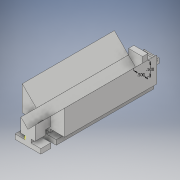
# Autodesk Inventor part: structureholder
Saved by Autodesk Inventor 2018 (Build 220112000, 112)
## iProperties
Created: 2019-02-25
Part Number: structureholder
Material: Generic
Document SubType Name: Modeling
Designer: F8PLTW
Density: 1 g/cm^3
Appearance: Default
Author: F8PLTW
Autodesk Inventor part; units mm, degrees
ref_plane "YZ Plane" through (0, 0, 0) normal (1, 0, 0) x (0, 1, 0)
ref_plane "XZ Plane" through (0, 0, 0) normal (0, 1, 0) x (-1, 0, 0)
ref_plane "XY Plane" through (0, 0, 0) normal (0, 0, 1) x (1, 0, 0)
sketch "Sketch1" plane through (0, 0, 0) normal (0, 0, 1) x (1, 0, 0)
  line L0 (-11.300905, 6.75881) -> (1.399095, 6.75881)
  line L1 (1.399095, 6.75881) -> (1.399095, -5.94119)
  line L2 (1.399095, -5.94119) -> (-11.300905, -5.94119)
  line L3 (-11.300905, -5.94119) -> (-11.300905, 6.75881)
  line L4 (-11.300905, 6.75881) -> (-1.742504, 6.75881) construction
  line L5 (-11.300905, 6.75881) -> (-4.950905, 0.40881)
  line L6 (1.399095, 6.75881) -> (-4.950905, 0.40881)
  point P0 (0, 0)
  dimension "d0" = 12.7
  dimension "d1" = 12.7
  constraints: 14 end point, 2 horizontal, 2 parallel, 1 perpendicular
  measures "d0" distance of L1.end L2.end
  measures "d1" distance of L0.end L1.end
sketch "Sketch1 outline for Extrusion1" plane through (0, 0, 0) normal (0, 0, 1) x (1, 0, 0)
  line L0 (-4.950905, 0.40881) -> (-11.300905, 6.75881)
  line L1 (1.399095, 6.75881) -> (-4.950905, 0.40881)
  line L2 (1.399095, -5.94119) -> (1.399095, 6.75881)
  line L3 (-11.300905, -5.94119) -> (1.399095, -5.94119)
  line L4 (-11.300905, 6.75881) -> (-11.300905, -5.94119)
extrude "Extrusion1" add sketch "Sketch1 outline for Extrusion1" along normal blind 101.6
sketch "Sketch1 outline for Extrusion2" plane through (0, 0, 0) normal (0, 0, 1) x (1, 0, 0)
  line L0 (1.399095, 6.75881) -> (-11.300905, 6.75881)
  line L1 (-4.950905, 0.40881) -> (1.399095, 6.75881)
  line L2 (-11.300905, 6.75881) -> (-4.950905, 0.40881)
extrude "Extrusion2" add sketch "Sketch1 outline for Extrusion2" along normal blind 5.08
sketch "Sketch2" plane through (-11.300905, 6.75881, 0) normal (0, 1, 0) x (1, 0, 0)
  line L0 (0, 0) -> (0, -101.6)
  line L1 (12.7, 0) -> (12.7, -101.6)
  line L2 (0, 0) -> (12.7, 0)
  line L3 (12.7, 0) -> (12.7, -5.078457)
  line L4 (12.7, -5.078457) -> (0, -5.078457)
  line L5 (0, -5.078457) -> (0, 0)
  point P0 (11.300905, 0)
  constraints: 8 end point, 2 parallel, 1 horizontal, 1 perpendicular, 1 point on line
sketch "Sketch2 outline for Extrusion3" plane through (-11.300905, 6.75881, 0) normal (0, 1, 0) x (1, 0, 0)
  line L0 (0, 0) -> (12.7, 0)
  line L1 (12.7, 0) -> (12.7, -5.078457)
  line L2 (12.7, -5.078457) -> (0, -5.078457)
  line L3 (0, -5.078457) -> (0, 0)
extrude "Extrusion3" add sketch "Sketch2 outline for Extrusion3" along normal blind 5.08
sketch "Sketch3" plane through (-11.300905, -5.94119, 0) normal (0, -1, 0) x (1, 0, 0)
  line L0 (12.7, 101.6) -> (6.35, 101.6) projected
  line L1 (0, 0) -> (12.7, 0) projected
  line L2 (9.4615, 101.6) -> (3.2385, 101.6)
  line L3 (3.2385, 101.6) -> (3.2385, 0)
  line L4 (3.2385, 0) -> (9.4615, 0)
  line L5 (9.4615, 0) -> (9.4615, 101.6)
  line L6 (6.35, 5.08) -> (6.35, 101.6) construction
  point P0 (11.300905, 0)
  dimension "d9" = 6.223
  constraints: 8 end point, 2 parallel, 2 point on line, 1 horizontal, 1 perpendicular, 1 other
  measures "d9" distance of L4.end L3.end
sketch "Sketch3 outline for Extrusion4" plane through (-11.300905, -5.94119, 0) normal (0, -1, 0) x (1, 0, 0)
  line L0 (9.4615, 0) -> (9.4615, 101.6)
  line L1 (3.2385, 0) -> (9.4615, 0)
  line L2 (3.2385, 101.6) -> (3.2385, 0)
  line L3 (9.4615, 101.6) -> (3.2385, 101.6)
extrude "Extrusion4" add sketch "Sketch3 outline for Extrusion4" along normal blind 7.3914
sketch "Sketch4" plane through (-1.839405, -5.94119, 101.6) normal (1, 0, 0) x (0, 0, -1)
  line L0 (101.6, -7.3914) -> (0, -7.3914) projected
  line L1 (101.6, 0) -> (101.6, -7.3914) projected
  line L2 (0, -7.3914) -> (101.6, -7.3914)
  line L3 (101.6, -7.3914) -> (101.6, -2.4384)
  line L4 (101.6, -2.4384) -> (0, -2.4384)
  line L5 (0, -2.4384) -> (0, -7.3914)
  point P0 (101.6, 5.94119)
  dimension "d12" = 4.953
  constraints: 8 end point, 2 parallel, 1 horizontal, 1 perpendicular, 1 point on line
  measures "d12" distance of L3.end L2.end
sketch "Sketch5" plane through (-8.062405, -5.94119, 0) normal (-1, 0, 0) x (0, 0, 1)
  line L0 (0, -7.3914) -> (101.6, -7.3914) projected
  line L1 (0, 0) -> (0, -7.3914) projected
  line L2 (101.6, -7.3914) -> (0, -7.3914)
  line L3 (0, -7.3914) -> (0, -2.4384)
  line L4 (0, -2.4384) -> (101.6, -2.4384)
  line L5 (101.6, -2.4384) -> (101.6, -7.3914)
  point P0 (0, 5.94119)
  dimension "d13" = 4.953
  constraints: 8 end point, 2 parallel, 1 horizontal, 1 perpendicular, 1 point on line
  measures "d13" distance of L2.end L3.end
sketch "Sketch5 outline for Extrusion5" plane through (-8.062405, -5.94119, 0) normal (-1, 0, 0) x (0, 0, 1)
  line L0 (0, -7.3914) -> (101.6, -7.3914)
  line L1 (0, -2.4384) -> (0, -7.3914)
  line L2 (101.6, -2.4384) -> (0, -2.4384)
  line L3 (101.6, -7.3914) -> (101.6, -2.4384)
extrude "Extrusion5" add sketch "Sketch5 outline for Extrusion5" along normal blind 8.763
sketch "Sketch4 outline for Extrusion6" plane through (-1.839405, -5.94119, 101.6) normal (1, 0, 0) x (0, 0, -1)
  line L0 (101.6, -7.3914) -> (101.6, -2.4384)
  line L1 (0, -7.3914) -> (101.6, -7.3914)
  line L2 (0, -2.4384) -> (0, -7.3914)
  line L3 (101.6, -2.4384) -> (0, -2.4384)
extrude "Extrusion6" add sketch "Sketch4 outline for Extrusion6" along normal blind 8.763
sketch "Sketch6" plane through (0, 0, 0) normal (0, 0, -1) x (-1, 0, 0)
  line L0 (-1.399095, -5.94119) -> (-1.399095, 6.75881)
  line L1 (-1.399095, 1.59881) -> (11.455496, 1.59881)
  line L2 (11.455496, 1.59881) -> (11.455496, -0.94119)
  line L3 (11.455496, -0.94119) -> (-1.399095, -0.94119)
  line L4 (-1.399095, -0.94119) -> (-1.399095, 1.59881)
  line L5 (11.300905, -5.94119) -> (8.062405, -5.94119)
  point P0 (0, 0)
  dimension "d18" = 2.54
  dimension "d19" = 5
  constraints: 8 end point, 2 parallel, 1 horizontal, 1 perpendicular, 1 point on line
  measures "d18" distance between parallel lines of L3 L1
  measures "d19" distance between parallel lines of L5 L3
sketch "Sketch6 outline for Extrusion7" plane through (0, 0, 0) normal (0, 0, -1) x (-1, 0, 0)
  line L0 (-1.399095, 1.59881) -> (11.455496, 1.59881)
  line L1 (11.455496, 1.59881) -> (11.455496, -0.94119)
  line L2 (11.455496, -0.94119) -> (-1.399095, -0.94119)
  line L3 (-1.399095, -0.94119) -> (-1.399095, 1.59881)
extrude "Extrusion7" add sketch "Sketch6 outline for Extrusion7" along normal blind 10
sketch "Sketch7" plane through (-11.300905, 1.59881, 0) normal (0, 1, 0) x (1, 0, 0)
  line L0 (-0.154591, 0) -> (-0.154591, 10)
  line L1 (12.7, 0) -> (12.7, 10)
  line L2 (-0.154591, 10) -> (12.7, 10)
  line L3 (12.7, 10) -> (12.7, 8.73819)
  line L4 (12.7, 8.73819) -> (-0.154591, 8.73819)
  line L5 (-0.154591, 8.73819) -> (-0.154591, 10)
  point P0 (11.300905, 0)
  constraints: 8 end point, 2 parallel, 1 horizontal, 1 perpendicular, 1 point on line
sketch "Sketch7 outline for Extrusion8" plane through (-11.300905, 1.59881, 0) normal (0, 1, 0) x (1, 0, 0)
  line L0 (-0.154591, 10) -> (12.7, 10)
  line L1 (12.7, 10) -> (12.7, 8.73819)
  line L2 (12.7, 8.73819) -> (-0.154591, 8.73819)
  line L3 (-0.154591, 8.73819) -> (-0.154591, 10)
extrude "Extrusion8" add sketch "Sketch7 outline for Extrusion8" along normal blind 2.5
fillet "Fillet1" radius 0.79375 2 edges at (-5.0282, 4.0988, -10) (-5.0282, 4.0988, -8.7382)
sketch "Sketch8" plane through (-11.300905, -13.33259, 0) normal (0, -1, 0) x (1, 0, 0)
  line L0 (18.2245, 101.6) -> (18.2245, 0)
  line L1 (-5.5245, 0) -> (-5.5245, 101.6)
  line L2 (18.2245, 92.457351) -> (-5.5245, 92.457351)
  line L3 (-5.5245, 92.457351) -> (-5.5245, 87.694851)
  line L4 (-5.5245, 87.694851) -> (18.2245, 87.694851)
  line L5 (18.2245, 87.694851) -> (18.2245, 92.457351)
  point P0 (11.300905, 0)
  dimension "d25" = 4.7625
  constraints: 8 end point, 2 parallel, 2 point on line, 1 horizontal, 1 perpendicular
  measures "d25" distance of L3.end L2.end
sketch "Sketch8 outline for Extrusion9" plane through (-11.300905, -13.33259, 0) normal (0, -1, 0) x (1, 0, 0)
  line L0 (18.2245, 87.694851) -> (18.2245, 92.457351)
  line L1 (-5.5245, 87.694851) -> (18.2245, 87.694851)
  line L2 (-5.5245, 92.457351) -> (-5.5245, 87.694851)
  line L3 (18.2245, 92.457351) -> (-5.5245, 92.457351)
extrude "Extrusion9" cut sketch "Sketch8 outline for Extrusion9" against normal blind 13.97
sketch "Sketch9" plane through (-11.300905, -13.33259, 0) normal (0, -1, 0) x (1, 0, 0)
  line L0 (-5.5245, 101.6) -> (18.2245, 101.6) projected
  line L1 (3.2385, 0) -> (-5.5245, 0) projected
  line L2 (18.2245, 101.6) -> (-5.5245, 101.6)
  line L3 (-5.5245, 101.6) -> (-5.5245, 0)
  line L4 (-5.5245, 0) -> (18.2245, 0)
  line L5 (18.2245, 0) -> (18.2245, 101.6)
  point P0 (11.300905, 0)
  constraints: 8 end point, 2 parallel, 1 horizontal, 1 perpendicular
sketch "Sketch9 outline for Extrusion10" plane through (-11.300905, -13.33259, 0) normal (0, -1, 0) x (1, 0, 0)
  line L0 (18.2245, 0) -> (18.2245, 101.6)
  line L1 (-5.5245, 0) -> (18.2245, 0)
  line L2 (-5.5245, 101.6) -> (-5.5245, 0)
  line L3 (18.2245, 101.6) -> (-5.5245, 101.6)
extrude "Extrusion10" cut sketch "Sketch9 outline for Extrusion10" against normal blind 0.127
sketch "Sketch10" plane through (-1.839405, -5.94119, 101.6) normal (0, -1, 0) x (1, 0, 0)
  line L0 (3.2385, -9.142649) -> (3.2385, 0)
  line L1 (0, -13.905149) -> (0, -101.6)
  line L2 (3.2385, 0) -> (0, 0)
  line L3 (0, 0) -> (0, -101.6)
  line L4 (0, -101.6) -> (3.2385, -101.6)
  line L5 (3.2385, -101.6) -> (3.2385, 0)
  line L6 (-9.4615, -9.142649) -> (-9.4615, 0)
  line L7 (-9.4615, -101.6) -> (3.2385, -101.6)
  line L8 (-9.4615, 0) -> (-5.941969, 0)
  line L9 (-5.941969, 0) -> (-5.941969, -101.6)
  line L10 (-5.941969, -101.6) -> (-9.4615, -101.6)
  line L11 (-9.4615, -101.6) -> (-9.4615, 0)
  point P0 (1.839405, -101.6)
  constraints: 16 end point, 4 parallel, 2 horizontal, 2 perpendicular, 1 point on line
sketch "Sketch10 outline for Extrusion11" plane through (-1.839405, -5.94119, 101.6) normal (0, -1, 0) x (1, 0, 0)
  line L0 (3.2385, -101.6) -> (3.2385, 0)
  line L1 (0, -101.6) -> (3.2385, -101.6)
  line L2 (0, 0) -> (0, -101.6)
  line L3 (3.2385, 0) -> (0, 0)
  line L4 (-9.4615, -101.6) -> (-5.941969, -101.6)
  line L5 (-9.4615, 0) -> (-9.4615, -101.6)
  line L6 (-5.941969, 0) -> (-9.4615, 0)
  line L7 (-5.941969, -101.6) -> (-5.941969, 0)
extrude "Extrusion11" cut sketch "Sketch10 outline for Extrusion11" against normal blind 0.127
sketch "Sketch11" plane through (6.923595, -5.94119, 101.6) normal (1, 0, 0) x (0, 0, -1)
  line L0 (0, -2.4384) -> (9.142649, -2.4384)
  line L1 (0, -2.4384) -> (101.6, -2.4384)
  line L2 (101.6, -2.4384) -> (101.6, -7.2644)
  line L3 (101.6, -7.2644) -> (0, -7.2644)
  line L4 (0, -7.2644) -> (0, -2.4384)
  point P0 (101.6, 5.94119)
  constraints: 8 end point, 2 parallel, 1 horizontal, 1 perpendicular
sketch "Sketch11 outline for Extrusion12" plane through (6.923595, -5.94119, 101.6) normal (1, 0, 0) x (0, 0, -1)
  line L0 (0, -2.4384) -> (101.6, -2.4384)
  line L1 (101.6, -2.4384) -> (101.6, -7.2644)
  line L2 (101.6, -7.2644) -> (0, -7.2644)
  line L3 (0, -7.2644) -> (0, -2.4384)
extrude "Extrusion12" cut sketch "Sketch11 outline for Extrusion12" against normal blind 0.0635
sketch "Sketch12" plane through (-16.825405, -5.94119, 0) normal (-1, 0, 0) x (0, 0, 1)
  line L0 (101.6, -7.2644) -> (101.6, -2.4384) projected
  line L1 (0, 0) -> (0, -2.4384) projected
  line L2 (101.6, -7.2644) -> (0, -7.2644)
  line L3 (0, -7.2644) -> (0, -2.4384)
  line L4 (0, -2.4384) -> (101.6, -2.4384)
  line L5 (101.6, -2.4384) -> (101.6, -7.2644)
  point P0 (0, 5.94119)
  constraints: 8 end point, 2 parallel, 1 horizontal, 1 perpendicular
sketch "Sketch12 outline for Extrusion13" plane through (-16.825405, -5.94119, 0) normal (-1, 0, 0) x (0, 0, 1)
  line L0 (101.6, -7.2644) -> (0, -7.2644)
  line L1 (0, -7.2644) -> (0, -2.4384)
  line L2 (0, -2.4384) -> (101.6, -2.4384)
  line L3 (101.6, -2.4384) -> (101.6, -7.2644)
extrude "Extrusion13" cut sketch "Sketch12 outline for Extrusion13" against normal blind 0.0635
sketch "Sketch13" plane through (-7.781374, -5.94119, 92.457351) normal (-1, 0, 0) x (0, 0, 1)
  line L0 (-92.457351, 0.127) -> (-4.7625, 0.127)
  line L1 (9.142649, -2.4384) -> (9.142649, 0.127)
  line L2 (-92.457351, 0.127) -> (9.142649, 0.127)
  line L3 (9.142649, 0.127) -> (9.142649, 0.002557)
  line L4 (9.142649, 0.002557) -> (-92.457351, 0.002557)
  line L5 (-92.457351, 0.002557) -> (-92.457351, 0.127)
  point P0 (-92.457351, 5.94119)
  constraints: 8 end point, 2 parallel, 1 horizontal, 1 perpendicular, 1 point on line
sketch "Sketch14" plane through (-7.781374, -5.94119, 0) normal (-1, 0, 0) x (0, 0, 1)
  line L0 (0, 0.127) -> (87.694851, 0.127)
  line L1 (92.457351, 0) -> (101.6, 0)
  line L2 (0, 0.127) -> (101.6, 0.127)
  line L3 (101.6, 0.127) -> (101.6, 0)
  line L4 (101.6, 0) -> (0, 0)
  line L5 (0, 0) -> (0, 0.127)
  point P0 (0, 5.94119)
  constraints: 8 end point, 2 parallel, 1 horizontal, 1 perpendicular
sketch "Sketch14 outline for Extrusion14" plane through (-7.781374, -5.94119, 0) normal (-1, 0, 0) x (0, 0, 1)
  line L0 (0, 0.127) -> (101.6, 0.127)
  line L1 (101.6, 0.127) -> (101.6, 0)
  line L2 (101.6, 0) -> (0, 0)
  line L3 (0, 0) -> (0, 0.127)
extrude "Extrusion14" add sketch "Sketch14 outline for Extrusion14" along normal blind 0.28194
sketch "Sketch15" plane through (-1.839405, -8.37959, 87.694851) normal (1, 0, 0) x (0, 0, -1)
  line L0 (-4.7625, 2.5654) -> (-13.905149, 2.5654)
  line L1 (87.694851, 2.4384) -> (87.694851, 0)
  line L2 (-13.905149, 2.5654) -> (87.694851, 2.5654)
  line L3 (87.694851, 2.5654) -> (87.694851, 0)
  line L4 (87.694851, 0) -> (-13.905149, 0)
  line L5 (-13.905149, 0) -> (-13.905149, 2.5654)
  point P0 (87.694851, 8.37959)
  constraints: 8 end point, 2 parallel, 1 horizontal, 1 perpendicular
sketch "Sketch15 outline for Extrusion15" plane through (-1.839405, -8.37959, 87.694851) normal (1, 0, 0) x (0, 0, -1)
  line L0 (-13.905149, 2.5654) -> (87.694851, 2.5654)
  line L1 (87.694851, 2.5654) -> (87.694851, 0)
  line L2 (87.694851, 0) -> (-13.905149, 0)
  line L3 (-13.905149, 0) -> (-13.905149, 2.5654)
extrude "Extrusion15" cut sketch "Sketch15 outline for Extrusion15" against normal blind 0.0635
sketch "Sketch16" plane through (-8.062405, -8.37959, 0) normal (-1, 0, 0) x (0, 0, 1)
  line L0 (101.6, 2.5654) -> (92.457351, 2.5654)
  line L1 (0, -4.826) -> (0, 0)
  line L2 (101.6, 2.5654) -> (0, 2.5654)
  line L3 (0, 2.5654) -> (0, 0)
  line L4 (0, 0) -> (101.6, 0)
  line L5 (101.6, 0) -> (101.6, 2.5654)
  point P0 (0, 8.37959)
  constraints: 8 end point, 2 parallel, 1 horizontal, 1 perpendicular
sketch "Sketch16 outline for Extrusion16" plane through (-8.062405, -8.37959, 0) normal (-1, 0, 0) x (0, 0, 1)
  line L0 (101.6, 0) -> (101.6, 2.5654)
  line L1 (0, 0) -> (101.6, 0)
  line L2 (0, 2.5654) -> (0, 0)
  line L3 (101.6, 2.5654) -> (0, 2.5654)
extrude "Extrusion16" cut sketch "Sketch16 outline for Extrusion16" against normal blind 0.0635
sketch "Sketch17" plane through (-11.300905, 0.63741, 0) normal (0, -1, 0) x (1, 0, 0)
  point P0 (11.300905, 0)
sketch "Sketch18" plane through (6.860095, -8.37959, 101.6) normal (0, 1, 0) x (1, 0, 0)
  line L0 (0, 0) -> (0, 9.142649)
  line L1 (-8.763, 9.142649) -> (0, 9.142649)
  line L2 (0, 0) -> (-8.763, 0)
  line L3 (-8.763, 0) -> (-8.763, 9.142649)
  line L4 (-8.763, 9.142649) -> (0, 9.142649)
  line L5 (0, 9.142649) -> (0, 0)
  line L6 (-14.859, 0) -> (-23.622, 0)
  line L7 (-14.859, 9.142649) -> (-23.622, 9.142649)
  line L8 (-14.859, 0) -> (-23.622, 0)
  line L9 (-23.622, 0) -> (-23.622, 9.142649)
  line L10 (-23.622, 9.142649) -> (-14.859, 9.142649)
  line L11 (-14.859, 9.142649) -> (-14.859, 0)
  line L12 (-8.763, 13.905149) -> (0, 13.905149)
  line L13 (-5.461, 101.6) -> (-18.161, 101.6)
  line L14 (0, 13.905149) -> (-8.763, 13.905149)
  line L15 (-8.763, 13.905149) -> (-8.763, 101.6)
  line L16 (-8.763, 101.6) -> (0, 101.6)
  line L17 (0, 101.6) -> (0, 13.905149)
  line L18 (-23.622, 13.905149) -> (-14.859, 13.905149)
  line L19 (-14.923409, 101.6) -> (-14.923409, 13.905149)
  line L20 (-23.622, 13.905149) -> (-14.923409, 13.905149)
  line L21 (-14.923409, 13.905149) -> (-14.923409, 101.6)
  line L22 (-14.923409, 101.6) -> (-23.622, 101.6)
  line L23 (-23.622, 101.6) -> (-23.622, 13.905149)
  point P0 (-6.860095, 101.6)
  constraints: 32 end point, 8 parallel, 4 horizontal, 4 perpendicular, 2 point on line
sketch "Sketch18 outline for Extrusion17" plane through (6.860095, -8.37959, 101.6) normal (0, 1, 0) x (1, 0, 0)
  line L0 (-8.763, 0) -> (0, 0)
  line L1 (-8.763, 9.142649) -> (-8.763, 0)
  line L2 (0, 9.142649) -> (-8.763, 9.142649)
  line L3 (0, 0) -> (0, 9.142649)
  line L4 (-14.859, 0) -> (-23.622, 0)
  line L5 (-23.622, 0) -> (-23.622, 9.142649)
  line L6 (-23.622, 9.142649) -> (-14.859, 9.142649)
  line L7 (-14.859, 9.142649) -> (-14.859, 0)
  line L8 (-14.923409, 13.905149) -> (-14.923409, 101.6)
  line L9 (-23.622, 13.905149) -> (-14.923409, 13.905149)
  line L10 (-23.622, 101.6) -> (-23.622, 13.905149)
  line L11 (-14.923409, 101.6) -> (-23.622, 101.6)
  line L12 (-8.763, 13.905149) -> (0, 13.905149)
  line L13 (-8.763, 101.6) -> (-8.763, 13.905149)
  line L14 (0, 101.6) -> (-8.763, 101.6)
  line L15 (0, 13.905149) -> (0, 101.6)
extrude "Extrusion17" cut sketch "Sketch18 outline for Extrusion17" against normal blind 0.508
sketch "Sketch19" plane through (6.860095, -5.94119, 101.6) normal (1, 0, 0) x (0, 0, -1)
  line L0 (0, 0.127) -> (0, -2.9464)
  line L1 (13.905149, -7.2644) -> (101.6, -7.2644)
  line L2 (0, -2.9464) -> (101.6, -2.9464)
  line L3 (101.6, -2.9464) -> (101.6, -7.2644)
  line L4 (101.6, -7.2644) -> (0, -7.2644)
  line L5 (0, -7.2644) -> (0, -2.9464)
  point P0 (101.6, 5.94119)
  constraints: 8 end point, 2 parallel, 1 horizontal, 1 perpendicular
sketch "Sketch19 outline for Extrusion18" plane through (6.860095, -5.94119, 101.6) normal (1, 0, 0) x (0, 0, -1)
  line L0 (0, -2.9464) -> (101.6, -2.9464)
  line L1 (101.6, -2.9464) -> (101.6, -7.2644)
  line L2 (101.6, -7.2644) -> (0, -7.2644)
  line L3 (0, -7.2644) -> (0, -2.9464)
extrude "Extrusion18" cut sketch "Sketch19 outline for Extrusion18" against normal blind 0.254
sketch "Sketch20" plane through (-16.761905, -5.94119, 0) normal (-1, 0, 0) x (0, 0, 1)
  line L0 (87.694851, -2.9464) -> (0, -2.9464)
  line L1 (101.6, -7.2644) -> (92.457351, -7.2644)
  line L2 (0, -2.9464) -> (101.6, -2.9464)
  line L3 (101.6, -2.9464) -> (101.6, -7.2644)
  line L4 (101.6, -7.2644) -> (0, -7.2644)
  line L5 (0, -7.2644) -> (0, -2.9464)
  point P0 (0, 5.94119)
  constraints: 8 end point, 2 parallel, 1 horizontal, 1 perpendicular
sketch "Sketch20 outline for Extrusion19" plane through (-16.761905, -5.94119, 0) normal (-1, 0, 0) x (0, 0, 1)
  line L0 (0, -2.9464) -> (101.6, -2.9464)
  line L1 (101.6, -2.9464) -> (101.6, -7.2644)
  line L2 (101.6, -7.2644) -> (0, -7.2644)
  line L3 (0, -7.2644) -> (0, -2.9464)
extrude "Extrusion19" cut sketch "Sketch20 outline for Extrusion19" against normal blind 0.254
sketch "Sketch21" plane through (-11.300905, 6.75881, 5.08) normal (-1, 0, 0) x (0, 0, 1)
  line L0 (82.614851, -12.573) -> (-5.08, -12.573)
  line L1 (96.52, -12.573) -> (96.52, -15.6464)
  line L2 (-5.08, -12.573) -> (96.52, -12.573)
  line L3 (96.52, -12.573) -> (96.52, -15.6464)
  line L4 (96.52, -15.6464) -> (-5.08, -15.6464)
  line L5 (-5.08, -15.6464) -> (-5.08, -12.573)
  point P0 (-5.08, -6.75881)
  constraints: 8 end point, 2 parallel, 1 horizontal, 1 perpendicular
sketch "Sketch21 outline for Extrusion20" plane through (-11.300905, 6.75881, 5.08) normal (-1, 0, 0) x (0, 0, 1)
  line L0 (-5.08, -12.573) -> (96.52, -12.573)
  line L1 (96.52, -12.573) -> (96.52, -15.6464)
  line L2 (96.52, -15.6464) -> (-5.08, -15.6464)
  line L3 (-5.08, -15.6464) -> (-5.08, -12.573)
extrude "Extrusion20" cut sketch "Sketch21 outline for Extrusion20" against normal blind 3.302
sketch "Sketch22" plane through (-1.902905, -8.37959, 87.694851) normal (1, 0, 0) x (0, 0, -1)
  line L0 (0, 2.5654) -> (87.694851, 2.5654)
  line L1 (-4.7625, -0.508) -> (-13.905149, -0.508)
  line L2 (87.694851, 2.5654) -> (-13.905149, 2.5654)
  line L3 (-13.905149, 2.5654) -> (-13.905149, -0.508)
  line L4 (-13.905149, -0.508) -> (87.694851, -0.508)
  line L5 (87.694851, -0.508) -> (87.694851, 2.5654)
  point P0 (87.694851, 8.37959)
  constraints: 8 end point, 2 parallel, 1 horizontal, 1 perpendicular
sketch "Sketch22 outline for Extrusion21" plane through (-1.902905, -8.37959, 87.694851) normal (1, 0, 0) x (0, 0, -1)
  line L0 (87.694851, -0.508) -> (87.694851, 2.5654)
  line L1 (-13.905149, -0.508) -> (87.694851, -0.508)
  line L2 (-13.905149, 2.5654) -> (-13.905149, -0.508)
  line L3 (87.694851, 2.5654) -> (-13.905149, 2.5654)
extrude "Extrusion21" cut sketch "Sketch22 outline for Extrusion21" against normal blind 0.254
sketch "Sketch23" plane through (-7.998905, -8.37959, 0) normal (-1, 0, 0) x (0, 0, 1)
  line L0 (87.694851, 2.5654) -> (0, 2.5654)
  line L1 (0, 2.5654) -> (101.6, 2.5654)
  line L2 (101.6, 2.5654) -> (101.6, -0.508)
  line L3 (101.6, -0.508) -> (0, -0.508)
  line L4 (0, -0.508) -> (0, 2.5654)
  point P0 (0, 8.37959)
  constraints: 8 end point, 2 parallel, 1 horizontal, 1 perpendicular
sketch "Sketch23 outline for Extrusion22" plane through (-7.998905, -8.37959, 0) normal (-1, 0, 0) x (0, 0, 1)
  line L0 (0, 2.5654) -> (101.6, 2.5654)
  line L1 (101.6, 2.5654) -> (101.6, -0.508)
  line L2 (101.6, -0.508) -> (0, -0.508)
  line L3 (0, -0.508) -> (0, 2.5654)
extrude "Extrusion22" cut sketch "Sketch23 outline for Extrusion22" against normal blind 0.254
sketch "Sketch24" plane through (1.399095, 6.75881, 101.6) normal (1, 0, 0) x (0, 0, -1)
  point P0 (101.6, -6.75881)
sketch "Sketch25" plane through (0, 0, 5.08) normal (0, 0, 1) x (1, 0, 0)
  line L0 (1.399095, 6.75881) -> (-4.950905, 0.40881)
  line L1 (-4.950905, 0.40881) -> (-25.57382, 21.031726)
  line L2 (-25.57382, 21.031726) -> (15.67201, 21.031726)
  line L3 (15.67201, 21.031726) -> (-4.950905, 0.40881)
  point P0 (0, 0)
  constraints: 6 end point, 1 collinear, 1 horizontal, 1 perpendicular
sketch "Sketch26" plane through (1.399095, 6.75881, 101.6) normal (1, 0, 0) x (0, 0, -1)
  line L0 (101.6, -12.573) -> (13.905149, -12.573)
  line L1 (13.905149, -12.573) -> (96.533031, -12.573)
  line L2 (96.533031, -12.573) -> (96.533031, 14.285186)
  line L3 (96.533031, 14.285186) -> (13.905149, 14.285186)
  line L4 (13.905149, 14.285186) -> (13.905149, -12.573)
  point P0 (101.6, -6.75881)
  constraints: 8 end point, 2 parallel, 1 horizontal, 1 perpendicular
sketch "Sketch26 outline for Extrusion23" plane through (1.399095, 6.75881, 101.6) normal (1, 0, 0) x (0, 0, -1)
  line L0 (13.905149, 14.285186) -> (13.905149, -12.573)
  line L1 (96.533031, 14.285186) -> (13.905149, 14.285186)
  line L2 (96.533031, -12.573) -> (96.533031, 14.285186)
  line L3 (13.905149, -12.573) -> (96.533031, -12.573)
extrude "Extrusion23" add sketch "Sketch26 outline for Extrusion23" against normal blind 12.7
sketch "Sketch27" plane through (1.399095, 1.59881, 0) normal (1, 0, 0) x (0, 0, -1)
  line L0 (-87.694851, 19.445186) -> (-87.694851, 5.16)
  line L1 (-87.694851, 19.445186) -> (-4.828406, 19.445186)
  line L2 (-4.828406, 19.445186) -> (-4.828406, -4.791789)
  line L3 (-4.828406, -4.791789) -> (-87.694851, -4.791789)
  line L4 (-87.694851, -4.791789) -> (-87.694851, 19.445186)
  point P0 (0, -1.59881)
  constraints: 8 end point, 2 parallel, 1 horizontal, 1 perpendicular
sketch "Sketch27 outline for Extrusion24" plane through (1.399095, 1.59881, 0) normal (1, 0, 0) x (0, 0, -1)
  line L0 (-87.694851, 19.445186) -> (-4.828406, 19.445186)
  line L1 (-4.828406, 19.445186) -> (-4.828406, -4.791789)
  line L2 (-4.828406, -4.791789) -> (-87.694851, -4.791789)
  line L3 (-87.694851, -4.791789) -> (-87.694851, 19.445186)
extrude "Extrusion24" add sketch "Sketch27 outline for Extrusion24" along normal blind 12.7
sketch "Sketch28" plane through (-11.300905, 1.59881, 0) normal (-1, 0, 0) x (0, 0, 1)
  line L0 (87.694851, 19.445186) -> (5.066969, 19.445186)
  line L1 (4.828406, 10.24) -> (4.828406, -4.791789)
  line L2 (87.694851, 19.445186) -> (4.828406, 19.445186)
  line L3 (4.828406, 19.445186) -> (4.828406, -4.791789)
  line L4 (4.828406, -4.791789) -> (87.694851, -4.791789)
  line L5 (87.694851, -4.791789) -> (87.694851, 19.445186)
  point P0 (0, -1.59881)
  constraints: 8 end point, 2 parallel, 1 horizontal, 1 perpendicular
sketch "Sketch28 outline for Extrusion25" plane through (-11.300905, 1.59881, 0) normal (-1, 0, 0) x (0, 0, 1)
  line L0 (87.694851, -4.791789) -> (87.694851, 19.445186)
  line L1 (4.828406, -4.791789) -> (87.694851, -4.791789)
  line L2 (4.828406, 19.445186) -> (4.828406, -4.791789)
  line L3 (87.694851, 19.445186) -> (4.828406, 19.445186)
extrude "Extrusion25" add sketch "Sketch28 outline for Extrusion25" along normal blind 12.7
sketch "Sketch25 outline for Extrusion26" plane through (0, 0, 5.08) normal (0, 0, 1) x (1, 0, 0)
  line L0 (-4.950905, 0.40881) -> (-25.57382, 21.031726)
  line L1 (-25.57382, 21.031726) -> (15.67201, 21.031726)
  line L2 (15.67201, 21.031726) -> (-4.950905, 0.40881)
extrude "Extrusion26" cut sketch "Sketch25 outline for Extrusion26" along normal blind 101.6
sketch "Sketch29" plane through (1.399095, 21.043996, 4.828406) normal (0, 1, 0) x (1, 0, 0)
  line L0 (-25.4, 0) -> (12.7, 0)
  line L1 (12.7, 0) -> (12.7, -82.866444)
  line L2 (12.7, -82.866444) -> (-25.4, -82.866444)
  line L3 (-25.4, -82.866444) -> (-25.4, 0)
  point P0 (-1.399095, 4.828406)
  constraints: 8 end point, 2 parallel, 1 horizontal, 1 perpendicular
sketch "Sketch29 outline for Extrusion27" plane through (1.399095, 21.043996, 4.828406) normal (0, 1, 0) x (1, 0, 0)
  line L0 (-25.4, 0) -> (12.7, 0)
  line L1 (12.7, 0) -> (12.7, -82.866444)
  line L2 (12.7, -82.866444) -> (-25.4, -82.866444)
  line L3 (-25.4, -82.866444) -> (-25.4, 0)
extrude "Extrusion27" cut sketch "Sketch29 outline for Extrusion27" against normal blind 1.27
sketch "Sketch30" plane through (-11.300905, -3.192978, 4.828406) normal (0, 0, -1) x (-1, 0, 0)
  line L0 (0, 15.031789) -> (0, 4.791789)
  line L1 (0, 9.911789) -> (12.7, 22.611789)
  line L2 (12.7, 0) -> (12.7, 22.651789)
  line L3 (0, 9.911789) -> (17.960512, 9.911789) construction
  line L4 (12.7, 22.611789) -> (19.140166, 29.051955)
  line L5 (-12.7, 4.791789) -> (-12.7, 15.031789)
  line L6 (-12.7, 9.911789) -> (-28.620083, 25.831872)
  line L7 (-12.7, 9.911789) -> (9.814397, 9.911789) construction
  line L8 (-28.620083, 25.831872) -> (-31.840166, 29.051955)
  line L9 (-31.840166, 29.051955) -> (19.140166, 29.051955)
  line L10 (-25.4, 0) -> (-25.4, 22.966975)
  line L11 (-12.7, 9.951789) -> (-6.35, 3.601789)
  line L12 (-12.7, 9.911789) -> (-6.35, 3.601789)
  line L13 (-6.35, 3.601789) -> (0, 9.951789)
  line L14 (-6.35, 3.601789) -> (0, 9.951789)
  point P0 (-11.300905, 3.192978)
  dimension "d64" = 45
  dimension "d65" = 135
  constraints: 18 end point, 3 point on line, 2 equal length, 2 horizontal, 2 midpoint, 1 perpendicular
  measures "d64" angle of L3 L1
  measures "d65" angle of L7 L6
sketch "Sketch30 outline for Extrusion28" plane through (-11.300905, -3.192978, 4.828406) normal (0, 0, -1) x (-1, 0, 0)
  line L0 (0, 9.951789) -> (0, 9.911789)
  line L1 (-6.35, 3.601789) -> (0, 9.951789)
  line L2 (-12.7, 9.951789) -> (-6.35, 3.601789)
  line L3 (-12.7, 9.911789) -> (-12.7, 9.951789)
  line L4 (-28.620083, 25.831872) -> (-12.7, 9.911789)
  line L5 (-31.840166, 29.051955) -> (-28.620083, 25.831872)
  line L6 (19.140166, 29.051955) -> (-31.840166, 29.051955)
  line L7 (12.7, 22.611789) -> (19.140166, 29.051955)
  line L8 (0, 9.911789) -> (12.7, 22.611789)
extrude "Extrusion28" cut sketch "Sketch30 outline for Extrusion28" against normal blind 152.4
sketch "Sketch31" plane through (1.399095, 1.59881, 0) normal (1, 0, 0) x (0, 0, -1)
  line L0 (-92.457351, -0.9614) -> (-92.457351, -7.413)
  line L1 (-87.694851, -10.4864) -> (-87.694851, -7.413)
  line L2 (-92.457351, -4.418125) -> (-87.694851, -4.418125)
  line L3 (-87.694851, -4.418125) -> (-87.694851, -9.88761)
  line L4 (-87.694851, -9.88761) -> (-92.457351, -9.88761)
  line L5 (-92.457351, -9.88761) -> (-92.457351, -4.418125)
  point P0 (0, -1.59881)
  constraints: 8 end point, 2 parallel, 2 point on line, 1 horizontal, 1 perpendicular
sketch "Sketch31 outline for Extrusion29" plane through (1.399095, 1.59881, 0) normal (1, 0, 0) x (0, 0, -1)
  line L0 (-92.457351, -4.418125) -> (-87.694851, -4.418125)
  line L1 (-87.694851, -4.418125) -> (-87.694851, -9.88761)
  line L2 (-87.694851, -9.88761) -> (-92.457351, -9.88761)
  line L3 (-92.457351, -9.88761) -> (-92.457351, -4.418125)
extrude "Extrusion29" cut sketch "Sketch31 outline for Extrusion29" against normal blind 50.8
sketch "Sketch32" plane through (-11.300905, 0.63741, 0) normal (0, -1, 0) x (1, 0, 0)
  line L0 (12.7, 87.694851) -> (6.5786, 87.694851)
  line L1 (6.5786, 92.457351) -> (12.7, 92.457351)
  line L2 (12.7, 87.694851) -> (6.5786, 87.694851)
  line L3 (6.5786, 87.694851) -> (6.5786, 92.457351)
  line L4 (6.5786, 92.457351) -> (12.7, 92.457351)
  line L5 (12.7, 92.457351) -> (12.7, 87.694851)
  line L6 (6.1214, 87.694851) -> (0, 87.694851)
  line L7 (0, 4.828406) -> (0, 101.6)
  line L8 (6.1214, 87.694851) -> (0, 87.694851)
  line L9 (0, 87.694851) -> (0, 92.457351)
  line L10 (0, 92.457351) -> (6.1214, 92.457351)
  line L11 (6.1214, 92.457351) -> (6.1214, 87.694851)
  point P0 (11.300905, 0)
  constraints: 16 end point, 4 parallel, 2 horizontal, 2 perpendicular, 2 point on line
sketch "Sketch32 outline for Extrusion30" plane through (-11.300905, 0.63741, 0) normal (0, -1, 0) x (1, 0, 0)
  line L0 (12.7, 87.694851) -> (6.5786, 87.694851)
  line L1 (6.5786, 87.694851) -> (6.5786, 92.457351)
  line L2 (6.5786, 92.457351) -> (12.7, 92.457351)
  line L3 (12.7, 92.457351) -> (12.7, 87.694851)
  line L4 (0, 87.694851) -> (6.1214, 87.694851)
  line L5 (0, 92.457351) -> (0, 87.694851)
  line L6 (6.1214, 92.457351) -> (0, 92.457351)
  line L7 (6.1214, 87.694851) -> (6.1214, 92.457351)
extrude "Extrusion30" add sketch "Sketch32 outline for Extrusion30" along normal blind 2.032
body "Solid1"
